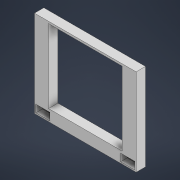
# Autodesk Inventor part: Circle_TestFit_V1
Saved by Autodesk Inventor 2022 (Build 260153000, 153)
## iProperties
Created: 2023-05-10
Part Number: Circle_TestFit_V1
Material: Generic
Document SubType Name: Modeling
Designer: Karl Spiteri
Density: 1 g/cm^3
Appearance: Default
Author: Karl Spiteri
Autodesk Inventor part; units mm, degrees
ref_plane "YZ Plane" through (0, 0, 0) normal (1, 0, 0) x (0, 1, 0)
ref_plane "XZ Plane" through (0, 0, 0) normal (0, 1, 0) x (-1, 0, 0)
ref_plane "XY Plane" through (0, 0, 0) normal (0, 0, 1) x (1, 0, 0)
sketch "Sketch4" plane through (0, 0, 0) normal (0, 0, 1) x (1, 0, 0)
  line L0 (0, 0) -> (-76, 0)
  line L1 (-76, 0) -> (-76, 65)
  line L2 (-76, 65) -> (0, 65)
  line L3 (0, 65) -> (0, 0)
  line L4 (-1, 1) -> (-11.6, 1)
  line L5 (-11.6, 1) -> (-11.6, 6.6)
  line L6 (-11.6, 6.6) -> (-1, 6.6)
  line L7 (-1, 6.6) -> (-1, 1)
  line L8 (-10.5, 63.5) -> (-65.5, 63.5)
  line L9 (-65.5, 63.5) -> (-65.5, 8.5)
  line L10 (-65.5, 8.5) -> (-10.5, 8.5)
  line L11 (-10.5, 8.5) -> (-10.5, 63.5)
  line L12 (-75, 1) -> (-64.4, 1)
  line L13 (-64.4, 1) -> (-64.4, 6.6)
  line L14 (-64.4, 6.6) -> (-75, 6.6)
  line L15 (-75, 6.6) -> (-75, 1)
  dimension "d26" = 76
  dimension "d27" = 65
  dimension "d36" = 10.6
  dimension "d37" = 5.6
  dimension "d40" = 55
  dimension "d41" = 55
  dimension "d42" = 10.6
  dimension "d43" = 5.6
  constraints: 32 end point, 8 parallel, 4 horizontal, 4 perpendicular
  measures "d26" distance of L1.end L2.end
  measures "d27" distance of L0.end L1.end
  measures "d36" distance of L5.end L6.end
  measures "d37" distance of L4.end L5.end
  measures "d40" distance of L10.end L9.end
  measures "d41" distance of L9.end L8.end
  measures "d42" distance of L14.end L13.end
  measures "d43" distance of L13.end L12.end
extrude "Extrusion8" add sketch "Sketch4" along normal blind 7 contours L0 L1 L2 L3 | L4 L5 L6 L7 | L15 L14 L13 L12
sketch "Sketch6" plane through (0, 0, 7) normal (0, 0, 1) x (1, 0, 0)
  line L0 (-1, 1) -> (-11.6, 1)
  line L1 (-11.6, 1) -> (-11.6, 6.6)
  line L2 (-11.6, 6.6) -> (-1, 6.6)
  line L3 (-1, 6.6) -> (-1, 1)
  line L4 (-75, 1) -> (-64.4, 1)
  line L5 (-64.4, 1) -> (-64.4, 6.6)
  line L6 (-64.4, 6.6) -> (-75, 6.6)
  line L7 (-75, 6.6) -> (-75, 1)
  point P0 (0, 0)
  dimension "d48" = 10.6
  dimension "d49" = 5.6
  dimension "d50" = 10.6
  dimension "d51" = 5.6
  constraints: 16 end point, 4 parallel, 2 horizontal, 2 perpendicular
  measures "d48" distance of L1.end L2.end
  measures "d49" distance of L0.end L1.end
  measures "d50" distance of L6.end L5.end
  measures "d51" distance of L5.end L4.end
extrude "Extrusion9" cut sketch "Sketch6" against normal blind 5
body "Solid5"
